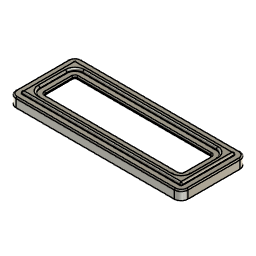
lcd_cover_v2 (Autodesk Fusion 360 design; units mm, degrees)
Autodesk Fusion 360 part; units mm, degrees
sketch "Sketch1" plane through (0, 0, 0) normal (0, 0, 1) x (1, 0, 0)
  line L0 (-1, 0) -> (-71, 0)
  line L1 (-72, -1) -> (-72, -24)
  line L2 (-71, -25) -> (-1, -25)
  line L3 (0, -24) -> (0, -1)
  arc A0 (-1, -25) -> (0, -24) centre (-1, -24) ccw
  arc A1 (-72, -24) -> (-71, -25) centre (-71, -24) ccw
  arc A2 (-71, 0) -> (-72, -1) centre (-71, -1) ccw
  arc A3 (0, -1) -> (-1, 0) centre (-1, -1) ccw
  line L4 (2, -24) -> (2, -1)
  arc A4 (2, -1) -> (-1, 2) centre (-1, -1) ccw
  line L5 (-1, 2) -> (-71, 2)
  arc A5 (-71, 2) -> (-74, -1) centre (-71, -1) ccw
  line L6 (-74, -1) -> (-74, -24)
  arc A6 (-74, -24) -> (-71, -27) centre (-71, -24) ccw
  line L7 (-71, -27) -> (-1, -27)
  arc A7 (-1, -27) -> (2, -24) centre (-1, -24) ccw
  point P0 (-72, 0)
  point P1 (0, -25)
  dimension "d1" = 72
  dimension "d2" = 25
  dimension "d3" = 1
  dimension "d4" = 2
  constraint horizontal L0
  constraint vertical L1
  constraint horizontal L2
  constraint vertical L3
  constraint coincident P1 L2
  constraint coincident P1 L3
  constraint tangent L2 A0
  constraint tangent L3 A0
  constraint tangent L1 A1
  constraint tangent L2 A1
  constraint equal A0 A1
  constraint coincident P0 L0
  constraint coincident P0 L1
  constraint tangent L0 A2
  constraint tangent L1 A2
  constraint equal A0 A2
  constraint coincident origin L0
  constraint coincident origin L3
  constraint tangent L0 A3
  constraint tangent L3 A3
  constraint equal A0 A3
  measures "d1" distance of origin P0
  measures "d2" distance of origin P1
  measures "d3" radius of A0
extrude "Extrude1" add sketch "Sketch1" along normal blind 3
sketch "Sketch2" plane through (0, 0, 3) normal (0, 0, 1) x (-1, 0, 0)
  arc A0 (0, 1) -> (1, 0) centre (1, 1) ccw
  line L0 (0, 1) -> (0, 24)
  arc A1 (1, 25) -> (0, 24) centre (1, 24) ccw
  line L1 (1, 25) -> (71, 25)
  arc A2 (72, 24) -> (71, 25) centre (71, 24) ccw
  line L2 (72, 24) -> (72, 1)
  arc A3 (71, 0) -> (72, 1) centre (71, 1) ccw
  line L3 (71, 0) -> (1, 0)
  arc A4 (1, 27) -> (-2, 24) centre (1, 24) ccw
  line L4 (-2, 24) -> (-2, 1)
  arc A5 (-2, 1) -> (1, -2) centre (1, 1) ccw
  line L5 (1, -2) -> (71, -2)
  arc A6 (71, -2) -> (74, 1) centre (71, 1) ccw
  line L6 (74, 1) -> (74, 24)
  arc A7 (74, 24) -> (71, 27) centre (71, 24) ccw
  line L7 (71, 27) -> (1, 27)
  line L8 (71, 27) -> (1, 27)
  line L9 (6.5, 19.5) -> (65.5, 19.5)
  line L10 (5.5, 6.5) -> (5.5, 18.5)
  line L11 (65.5, 5.5) -> (6.5, 5.5)
  line L12 (66.5, 18.5) -> (66.5, 6.5)
  arc A8 (6.5, 19.5) -> (5.5, 18.5) centre (6.5, 18.5) ccw
  arc A9 (66.5, 18.5) -> (65.5, 19.5) centre (65.5, 18.5) ccw
  arc A10 (65.5, 5.5) -> (66.5, 6.5) centre (65.5, 6.5) ccw
  arc A11 (5.5, 6.5) -> (6.5, 5.5) centre (6.5, 6.5) ccw
  dimension "d8" = 1
  constraint tangent L9 A8
  constraint tangent L10 A8
  constraint tangent L9 A9
  constraint tangent L12 A9
  constraint equal A8 A9
  constraint tangent L11 A10
  constraint tangent L12 A10
  constraint equal A8 A10
  constraint tangent L10 A11
  constraint tangent L11 A11
  constraint equal A8 A11
  measures "d8" radius of A8
extrude "Extrude2" add sketch "Sketch2" along normal blind 1 contours A0 L0 A1 L1 A2 L2 A3 L3 | A4 L4 A5 L5 A6 L6 A7 L7 L8
fillet "Fillet1" radius 0.5 8 edges at (-66.5, -12.5, 4) (-66.2071, -5.7929, 4) (-36, -5.5, 4) (-5.7929, -5.7929, 4) (-5.5, -12.5, 4) (-5.7929, -19.2071, 4) (-36, -19.5, 4) (-66.2071, -19.2071, 4)
fillet "Fillet2" radius 0.5 8 edges at (-73.1213, 1.1213, 4) (-74, -12.5, 4) (-73.1213, -26.1213, 4) (-36, -27, 4) (1.1213, -26.1213, 4) (2, -12.5, 4) (1.1213, 1.1213, 4) (-36, 2, 4)
sketch "Sketch3" plane through (0, 0, 4) normal (0, 0, 1) x (-1, 0, 0)
  line L0 (67, 18.5) -> (67, 6.5)
  arc A0 (65.5, 5) -> (67, 6.5) centre (65.5, 6.5) ccw
  line L1 (65.5, 5) -> (6.5, 5)
  arc A1 (5, 6.5) -> (6.5, 5) centre (6.5, 6.5) ccw
  line L2 (5, 6.5) -> (5, 18.5)
  arc A2 (6.5, 20) -> (5, 18.5) centre (6.5, 18.5) ccw
  line L3 (6.5, 20) -> (65.5, 20)
  arc A3 (67, 18.5) -> (65.5, 20) centre (65.5, 18.5) ccw
  arc A4 (71, -1.5) -> (73.5, 1) centre (71, 1) ccw
  line L4 (73.5, 1) -> (73.5, 24)
  arc A5 (73.5, 24) -> (71, 26.5) centre (71, 24) ccw
  line L5 (71, 26.5) -> (1, 26.5)
  arc A6 (1, 26.5) -> (-1.5, 24) centre (1, 24) ccw
  line L6 (-1.5, 24) -> (-1.5, 1)
  arc A7 (-1.5, 1) -> (1, -1.5) centre (1, 1) ccw
  line L7 (1, -1.5) -> (71, -1.5)
  line L8 (0.5, 24) -> (0.5, 1)
  arc A8 (0.5, 1) -> (1, 0.5) centre (1, 1) ccw
  line L9 (1, 0.5) -> (71, 0.5)
  arc A9 (71, 0.5) -> (71.5, 1) centre (71, 1) ccw
  line L10 (71.5, 1) -> (71.5, 24)
  arc A10 (71.5, 24) -> (71, 24.5) centre (71, 24) ccw
  line L11 (71, 24.5) -> (1, 24.5)
  arc A11 (1, 24.5) -> (0.5, 24) centre (1, 24) ccw
  arc A12 (3, 6.5) -> (6.5, 3) centre (6.5, 6.5) ccw
  line L12 (65.5, 3) -> (6.5, 3)
  arc A13 (65.5, 3) -> (69, 6.5) centre (65.5, 6.5) ccw
  line L13 (69, 18.5) -> (69, 6.5)
  arc A14 (69, 18.5) -> (65.5, 22) centre (65.5, 18.5) ccw
  line L14 (6.5, 22) -> (65.5, 22)
  arc A15 (6.5, 22) -> (3, 18.5) centre (6.5, 18.5) ccw
  line L15 (3, 6.5) -> (3, 18.5)
  dimension "d15" = -2
  dimension "d16" = -2
extrude "Extrude3" add sketch "Sketch3" along normal blind 1 contours L8 A8 L9 A9 L10 A10 L11 A11
fillet "Fillet3" radius 0.75 16 edges at (-67.9749, -20.9749, 5) (-69, -12.5, 5) (-67.9749, -4.0251, 5) (-36, -3, 5) (-4.0251, -4.0251, 5) (-3, -12.5, 5) (-4.0251, -20.9749, 5) (-36, -22, 5) (-36, -0.5, 5) (-71.3536, -0.6464, 5) (-71.5, -12.5, 5) (-71.3536, -24.3536, 5) (-36, -24.5, 5) (-0.6464, -24.3536, 5) (-0.5, -12.5, 5) (-0.6464, -0.6464, 5)
